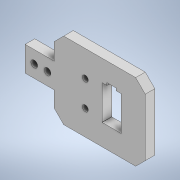
# Autodesk Inventor part: Servo Holder Module
Saved by Autodesk Inventor 2020 (Build 240168000, 168)
## iProperties
Created: 2020-03-03
Part Number: Servo Holder Module
Material: Generic
Document SubType Name: Modeling
Designer: Varun Kumar
Density: 1 g/cm^3
Appearance: Default
Author: Varun Kumar
Autodesk Inventor part; units mm, degrees
ref_plane "YZ Plane" through (0, 0, 0) normal (1, 0, 0) x (0, 1, 0)
ref_plane "XZ Plane" through (0, 0, 0) normal (0, 1, 0) x (-1, 0, 0)
ref_plane "XY Plane" through (0, 0, 0) normal (0, 0, 1) x (1, 0, 0)
sketch "Sketch1" plane through (0, 0, 0) normal (0, 0, 1) x (1, 0, 0)
  line L0 (-38.1, -25.4) -> (38.1, -25.4)
  line L1 (38.1, -25.4) -> (38.1, 25.4)
  line L2 (38.1, 25.4) -> (-38.1, 25.4)
  line L3 (-38.1, 25.4) -> (-38.1, -25.4)
  line L4 (-38.1, -25.4) -> (38.1, 25.4) construction
  line L5 (38.1, -25.4) -> (-38.1, 25.4) construction
  point P0 (0, 0)
  dimension "d0" = 76.2
  dimension "d1" = 50.8
  constraints: 12 end point, 2 midpoint, 2 parallel, 1 horizontal, 1 perpendicular
  measures "d0" distance of L2.end L1.end
  measures "d1" distance of L1.end L0.end
extrude "Extrusion1" add sketch "Sketch1" along normal blind 6.35
sketch "Sketch3" plane through (38.1, -25.4, 0) normal (1, 0, 0) x (0, 0, -1)
  line L0 (0, 0) -> (0, 50.8) projected
  line L1 (0, 50.8) -> (-6.35, 50.8) projected
  line L2 (-6.35, 0) -> (-6.35, 50.8) projected
  line L3 (0, 0) -> (-6.35, 0) projected
  point P0 (0, 25.4)
extrude "Extrusion3" cut sketch "Sketch3" against normal blind 15.875
sketch "Sketch4" plane through (-38.1, -25.4, 0) normal (-1, 0, 0) x (0, 0, 1)
  line L0 (6.35, 16.7952) -> (0, 16.7952)
  line L1 (0, 16.7952) -> (0, 33.2952)
  line L2 (0, 33.2952) -> (6.35, 33.2952)
  line L3 (6.35, 33.2952) -> (6.35, 16.7952)
  line L4 (6.35, 16.7952) -> (0, 33.2952) construction
  line L5 (0, 16.7952) -> (6.35, 33.2952) construction
  line L6 (6.35, 50.8) -> (6.35, 0) projected
  line L7 (6.35, 50.8) -> (3.175, 50.8)
  line L8 (0, 50.8) -> (6.35, 50.8) projected
  line L9 (3.175, 50.8) -> (3.175, 25.0452)
  point P0 (0, 25.4)
  dimension "d9" = 6.35
  dimension "d10" = 16.5
  constraints: 16 end point, 3 midpoint, 3 parallel, 1 horizontal, 1 perpendicular
  measures "d9" distance of L1.end L2.end
  measures "d10" distance of L0.end L1.end
extrude "Extrusion4" add sketch "Sketch4" along normal blind 3.302 contours L0 L1 L2 L3
chamfer "Chamfer1" distance 6.35 angle 45 4 edges at (-38.1, -25.4, 3.175) (-38.1, 25.4, 3.175) (22.225, -25.4, 3.175) (22.225, 25.4, 3.175)
sketch "Sketch6" plane through (0, 0, 6.35) normal (0, 0, 1) x (1, 0, 0)
  line L0 (5.9693, 11.0167) -> (6.0307, -10.9832) projected
  line L1 (-6.0307, 10.9832) -> (6.0307, 10.9832)
  line L2 (6.0307, 10.9832) -> (6.0307, -10.9832)
  line L3 (6.0307, -10.9832) -> (-6.0307, -10.9832)
  line L4 (-6.0307, -10.9832) -> (-6.0307, 10.9832)
  point P0 (0, 0)
  point P1 (5.9694, 10.9832)
  constraints: 8 end point, 2 parallel, 1 horizontal, 1 perpendicular
extrude "Extrusion5" cut sketch "Sketch6" against normal up to surface (6.35 mm away) contours L0 L3 L4 L1
sketch "Sketch7" plane through (0, 0, 6.35) normal (0, 0, 1) x (1, 0, 0)
  circle A0 centre (-17.4683, 8.1506) radius 2 projected
  circle A1 centre (-17.4683, -8.8674) radius 2 projected
  line L0 (-8.7307, -16.3858) -> (-26.0507, -16.3858) projected
  line L1 (-8.7307, -16.3858) -> (-8.7307, 15.669) projected
  line L2 (-8.7307, 15.669) -> (-26.0507, 15.669) projected
  line L3 (-26.0507, -16.3858) -> (-26.0507, 15.669) projected
  circle A2 centre (-17.4683, 8.1506) radius 2
  circle A3 centre (-17.4683, -8.8674) radius 2
  point P0 (0, 0)
  dimension "d21" = 4
  dimension "d22" = 4
  constraints: 2 centre point, 2 coincident
  measures "d21" diameter of A2
  measures "d22" diameter of A3
extrude "Extrusion6" cut sketch "Sketch7" against normal up to surface (6.35 mm away) contours A0 | A1
sketch "Sketch8" plane through (-41.402, -25.4, 0) normal (-1, 0, 0) x (0, 0, 1)
  line L0 (6.35, 16.7952) -> (6.35, 33.2952) projected
  line L1 (6.35, 33.2952) -> (0, 33.2952) projected
  line L2 (0, 33.2952) -> (0, 16.7952) projected
  line L3 (0, 16.7952) -> (6.35, 16.7952) projected
  line L4 (6.35, 16.7952) -> (6.35, 33.2952) projected
  line L5 (6.35, 33.2952) -> (0, 33.2952) projected
  line L6 (0, 33.2952) -> (0, 16.7952) projected
  line L7 (0, 16.7952) -> (6.35, 16.7952) projected
  point P0 (0, 25.4)
extrude "Extrusion7" add sketch "Sketch8" along normal blind 12.7
sketch "Sketch9" plane through (-38.1, -8.6048, 0) normal (0, 0, -1) x (1, 0, 0)
  line L0 (0, 0) -> (0, -16.5) projected
  line L1 (0, 0) -> (0, -8.25)
  line L2 (0, 0) -> (-16.002, 0) projected
  circle A0 centre (-4.3815, -8.25) radius 2.25
  circle A1 centre (-13.1445, -8.25) radius 2.25
  line L3 (0, -8.25) -> (-4.3815, -8.25)
  line L4 (-4.3815, -8.25) -> (-13.1445, -8.25)
  point P0 (38.1, -8.6048)
  dimension "d28" = 4.5
  dimension "d31" = 4.5
  dimension "d36" = 4.3815
  dimension "d37" = 8.763
  constraints: 6 end point, 2 centre point, 2 coincident, 1 midpoint, 1 perpendicular, 1 point on line
  measures "d28" diameter of A0
  measures "d31" diameter of A1
  measures "d36" distance of L1.end L3.end
  measures "d37" distance of L3.end L4.end
sketch "Sketch10" plane through (-54.102, -25.4, 0) normal (-1, 0, 0) x (0, 0, 1)
  line L0 (6.35, 16.7952) -> (6.35, 33.2952) projected
  line L1 (6.35, 33.2952) -> (0, 33.2952) projected
  line L2 (0, 33.2952) -> (0, 16.7952) projected
  line L3 (0, 16.7952) -> (6.35, 16.7952) projected
  point P0 (0, 25.4)
extrude "Extrusion8" add sketch "Sketch10" along normal blind 3.1877
extrude "Extrusion9" cut sketch "Sketch9" against normal up to surface (6.35 mm away)
sketch "Sketch11" plane through (0, 0, 6.35) normal (0, 0, 1) x (1, 0, 0)
  line L0 (-6.0307, 10.9832) -> (5.9694, 10.9832) projected
  line L1 (5.9694, 10.9832) -> (6.0307, -10.9832) projected
  line L2 (-6.0307, -10.9832) -> (-6.0307, 10.9832) projected
  line L3 (6.0307, -10.9832) -> (-6.0307, -10.9832) projected
  line L4 (6.2226, 11.2372) -> (-6.2847, 11.2372)
  line L5 (-6.2847, 11.2372) -> (-6.2847, -11.2372)
  line L6 (-6.2847, -11.2372) -> (6.2854, -11.2372)
  line L7 (6.2854, -11.2372) -> (6.2226, 11.2372)
  line L8 (6.2226, 11.2372) -> (-6.2847, 11.2372)
  line L9 (-6.2847, 11.2372) -> (-6.2847, 11.396)
  line L10 (-6.2847, 11.396) -> (6.2226, 11.396)
  line L11 (6.2226, 11.396) -> (6.2226, 11.2372)
  line L12 (6.2854, -11.2372) -> (-6.2876, -11.2372)
  line L13 (-6.2876, -11.2372) -> (-6.2876, -11.396)
  line L14 (-6.2876, -11.396) -> (6.2854, -11.396)
  line L15 (6.2854, -11.396) -> (6.2854, -11.2372)
  point P0 (0, 0)
  dimension "d38" = 0.254
  dimension "d41" = 0.1588
  dimension "d42" = 12.573
  dimension "d43" = 0.1588
  constraints: 24 end point, 4 parallel, 2 horizontal, 2 perpendicular, 3 other
  measures "d38" distance between parallel lines of L0 L4
  measures "d41" distance of L8.end L9.end
  measures "d42" distance of L14.end L13.end
  measures "d43" distance of L13.end L12.end
extrude "Extrusion10" cut sketch "Sketch11" against normal up to surface (6.35 mm away) contours L7 L6 L5 L4
sketch "Sketch12" plane through (0, 0, 6.35) normal (0, 0, 1) x (1, 0, 0)
  line L0 (6.2226, 11.2372) -> (-6.2847, 11.2372)
  line L1 (-6.2847, 11.2372) -> (-6.2847, -11.2372)
  line L2 (-6.2847, -11.2372) -> (6.2854, -11.2372)
  line L3 (6.2854, -11.2372) -> (6.2226, 11.2372)
  line L4 (6.2226, 11.2372) -> (-6.2847, 11.2372)
  line L5 (-6.2847, 11.2372) -> (-6.2847, 11.396)
  line L6 (-6.2847, 11.396) -> (6.2226, 11.396)
  line L7 (6.2226, 11.396) -> (6.2226, 11.2372)
  line L8 (6.2854, -11.2372) -> (-6.2876, -11.2372)
  line L9 (-6.2876, -11.2372) -> (-6.2876, -11.396)
  line L10 (-6.2876, -11.396) -> (6.2854, -11.396)
  line L11 (6.2854, -11.396) -> (6.2854, -11.2372)
  point P0 (0, 0)
  point P1 (-6.2847, 11.2372)
  dimension "d44" = 0.1588
  dimension "d45" = 12.573
  dimension "d46" = 0.1588
  constraints: 24 end point, 4 parallel, 2 horizontal, 2 perpendicular
  measures "d44" distance of L5.start L5.end
  measures "d45" distance of L10.end L9.end
  measures "d46" distance of L9.end L9.start
extrude "Extrusion11" cut sketch "Sketch12" against normal up to surface (6.35 mm away) contours L0 L5 L6 L7 | L11 L10 L9 L8 L2
sketch "Sketch13" plane through (0, 0, 6.35) normal (0, 0, 1) x (1, 0, 0)
  line L0 (-6.2847, 11.396) -> (-3.1097, 11.396)
  line L1 (-6.2847, 11.396) -> (6.2226, 11.396) projected
  line L2 (-6.2847, 11.396) -> (-3.1097, 11.396) construction
  line L3 (6.2226, 11.396) -> (3.0476, 11.396)
  line L4 (-3.1097, 11.396) -> (3.0476, 11.396)
  line L5 (3.0476, 11.396) -> (3.0476, 12.9835)
  line L6 (3.0476, 12.9835) -> (-3.1097, 12.9835)
  line L7 (-3.1097, 12.9835) -> (-3.1097, 11.396)
  point P0 (0, 0)
  dimension "d49" = 3.175
  dimension "d50" = 0
  dimension "d51" = 3.175
  dimension "d52" = 1.5875
  constraints: 14 end point, 2 collinear, 2 horizontal, 2 parallel, 1 perpendicular, 1 point on line
  measures "d49" distance of L0.start L0.end
  measures "d50" distance between parallel lines of L2 L0
  measures "d51" distance of L1.end L3.end
  measures "d52" distance of L5.end L4.end
extrude "Extrusion12" cut sketch "Sketch13" against normal up to surface (6.35 mm away)
body "Solid1"
